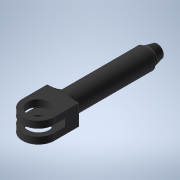
# Autodesk Inventor part: Push Rod v2
Saved by Autodesk Inventor 2022 (Build 260153000, 153)
## iProperties
Created: 2023-01-26
Part Number: Push Rod v2
Material: Generic
Document SubType Name: Modeling
Designer: ASUS
Density: 1 g/cm^3
Appearance: Default
Author: ASUS
Autodesk Inventor part; units mm, degrees
ref_plane "YZ Plane" through (0, 0, 0) normal (1, 0, 0) x (0, 1, 0)
ref_plane "XY Plane" through (0, 0, 0) normal (0, 0, 1) x (1, 0, 0)
sketch "Sketch1" plane through (0, 0, 0) normal (0, 1, 0) x (-1, 0, 0)
  circle A0 centre (0, 0) radius 11.05
  circle A1 centre (0, 0) radius 16
  line L0 (16, 0) -> (-16, 0)
  line L1 (-16, 0) -> (-16, -25)
  line L2 (-16, -25) -> (16, -25)
  line L3 (16, -25) -> (16, 0)
  dimension "d1" = 32
  dimension "d0" = 22.1
  dimension "d2" = 25
  constraints: 8 end point, 2 coincident, 2 parallel, 1 centre point, 1 horizontal, 1 perpendicular, 3 other
  measures "d0" diameter of A0
  measures "d2" distance of L0.end L1.end
extrude "Extrusion1" add sketch "Sketch1" along normal blind 21 contours L0 A1 A0 | A0 L0 A1 | L3 L2 L1 A1
sketch "Sketch2" plane through (16, 0, 0) normal (1, 0, 0) x (0, 0, -1)
  line L0 (-11, 14) -> (11, 14)
  line L1 (11, 14) -> (11, 7)
  line L2 (11, 7) -> (-11, 7)
  line L3 (-11, 7) -> (-11, 14)
  line L4 (0, 21) -> (25, 21) projected
  line L5 (-16, 0) -> (-16, 21) projected
  line L6 (-11, 14) -> (-16, 14)
  line L7 (-16, 14) -> (-16, 7)
  line L8 (-16, 7) -> (-11, 7)
  line L9 (-11, 7) -> (-11, 14)
  point P0 (0, 0)
  dimension "d5" = 22
  dimension "d6" = 11
  dimension "d7" = 7
  dimension "d8" = 7
  constraints: 16 end point, 4 parallel, 2 horizontal, 2 perpendicular, 1 point on line
  measures "d5" distance of L1.end L2.end
  measures "d6" distance from line of point (0, 0) L3
  measures "d7" distance of L0.end L1.end
  measures "d8" distance between parallel lines of L4 L0
extrude "Extrusion2" cut sketch "Sketch2" against normal through all
sketch "Sketch3" plane through (16, 7, 0) normal (0, 1, 0) x (1, 0, 0)
  circle A0 centre (-16, 0) radius 19.4165
  point P0 (-16, 0)
  point P1 (-32, 11)
  constraints: 1 coincident, 3 other
extrude "Extrusion3" cut sketch "Sketch3" along normal blind 7
ref_plane "Work Plane1" through (16, 0, -30) normal (0, 0, -1) x (-1, 0, 0)
sketch "Sketch4" plane through (16, 0, -30) normal (0, 0, -1) x (-1, 0, 0)
  circle A0 centre (16, 10.5) radius 10.5
  point P0 (16, 0)
  constraints: 1 centre point
loft "Loft1" add profiles "Sketch4" section 2 edges at (0, 0, -25) (-16, 10.5, -25) (0, 21, -25) (16, 10.5, -25)
sketch "Sketch5" plane through (0, 10.5, -30) normal (0, 0, -1) x (-1, 0, 0)
  circle A0 centre (0, 0) radius 10.5
  point P0 (0, -10.5)
  constraints: 1 centre point
extrude "Extrusion4" add sketch "Sketch5" along normal blind 61
sketch "Sketch6" plane through (0, 0, 0) normal (1, 0, 0) x (0, 1, 0)
  line L0 (21, -60) -> (21, -117)
  arc A0 (21, -108.5) -> (19, -112.5) centre (21, -111) ccw
  line L1 (21, -108.5) -> (21, -92.5)
  line L2 (17, -121) -> (4, -121)
  line L3 (10.5, -121) -> (10.5, -60)
  line L4 (21, -60) -> (0, -60)
  line L5 (19, -112.5) -> (17, -121)
  line L6 (21, -92.5) -> (21, -117)
  arc A1 (17, -121) -> (21, -117) centre (17, -117) ccw
  line L7 (0, -91) -> (21, -91) projected
  line L8 (21, -25) -> (21, 0) projected
  line L9 (21, 0) -> (21, -113.3676) construction
  point P0 (0, 0)
  point P1 (0, 0)
  dimension "d21" = 5
  dimension "d22" = 10
  dimension "d23" = 2
  dimension "d24" = 30
  dimension "d25" = 0
  dimension "d26" = 10.5
  dimension "d27" = 166.759
  constraints: 16 end point, 4 point on circle, 3 point on line, 2 centre point, 2 midpoint, 2 tangent, 2 vertical
  measures "d21" diameter of A0
  measures "d22" distance from line of L2 A0.centre
  measures "d23" distance from line of L5.start L0
  measures "d24" distance between parallel lines of L7 L2
  measures "d25" distance between parallel lines of L9 L0
  measures "d26" distance between parallel lines of L3 L0
  measures "d27" angle of L0 L5
revolve "Revolution1" add sketch "Sketch6" angle 360 about axis through (0, 10.5, -121) along (0, 0, 1) contours L0 L7 L3 L4 | L0 A0 L5 L2 L3 L7
sketch "Sketch7" plane through (0, 21, 0) normal (0, 1, 0) x (1, 0, 0)
  line L0 (-27.5417, 91) -> (29.185, 91)
  line L1 (29.185, 91) -> (29.185, -13.5)
  line L2 (29.185, -13.5) -> (-27.5417, -13.5)
  line L3 (-27.5417, -13.5) -> (-27.5417, 91)
  line L4 (6.5, 121) -> (-6.5, 121) projected
  point P0 (0, 0)
  dimension "d29" = 30
  dimension "d30" = 104.5
  constraints: 8 end point, 2 parallel, 1 horizontal, 1 perpendicular
  measures "d29" distance between parallel lines of L0 L4
  measures "d30" distance of L0.end L1.end
ref_plane "Work Plane2" through (0, 10.75, 0) normal (0, 1, 0) x (-1, 0, 0)
sketch "Sketch8" plane through (0, 10.75, 0) normal (0, 1, 0) x (-1, 0, 0)
  line L0 (-32.5, -91) -> (32.5, -91)
  line L1 (32.5, -91) -> (32.5, 69.4)
  line L2 (32.5, 69.4) -> (-32.5, 69.4)
  line L3 (-32.5, 69.4) -> (-32.5, -91)
  line L4 (-6.5, -121) -> (6.5, -121) projected
  line L5 (32.5, -66) -> (-32.5, -66)
  line L6 (32.5, -53.5) -> (-32.5, -53.5)
  circle A0 centre (0, 69.4) radius 32.5
  point P0 (0, 0)
  dimension "d32" = 65
  dimension "d33" = 30
  dimension "d34" = 160.4
  dimension "d35" = 32.5
  dimension "d36" = 25
  dimension "d37" = 12.5
  dimension "d38" = 65
  dimension "d39" = 0
  constraints: 12 end point, 4 point on line, 3 perpendicular, 2 parallel, 1 centre point, 1 horizontal
  measures "d32" distance of L1.end L2.end
  measures "d33" distance between parallel lines of L4 L0
  measures "d34" distance of L0.end L1.end
  measures "d35" distance from line of L1 point (0, 0)
  measures "d36" distance between parallel lines of L0 L5
  measures "d37" distance between parallel lines of L5 L6
  measures "d38" diameter of A0
  measures "d39" distance from line of L2 A0.centre
sketch "Sketch9" plane through (0, 0, 0) normal (1, 0, 0) x (0, 1, 0)
  line L0 (-22, -91) -> (43, -91)
  line L1 (43, -91) -> (43, 13.5)
  line L2 (43, 13.5) -> (-22, 13.5)
  line L3 (-22, 13.5) -> (-22, -91)
  line L4 (4, -121) -> (17, -121) projected
  point P0 (0, 0)
  point P1 (10.5, 0)
  dimension "d40" = 65
  dimension "d41" = 104.5
  dimension "d42" = 30
  dimension "d43" = 10.5
  dimension "d44" = 32.5
  constraints: 8 end point, 2 parallel, 1 horizontal, 1 perpendicular
  measures "d40" distance of L2.end L1.end
  measures "d41" distance of L0.end L1.end
  measures "d42" distance between parallel lines of L4 L0
  measures "d43" distance of point (10.5, 0) point (0, 0)
  measures "d44" distance from line of point (10.5, 0) L1
body "Solid1"
